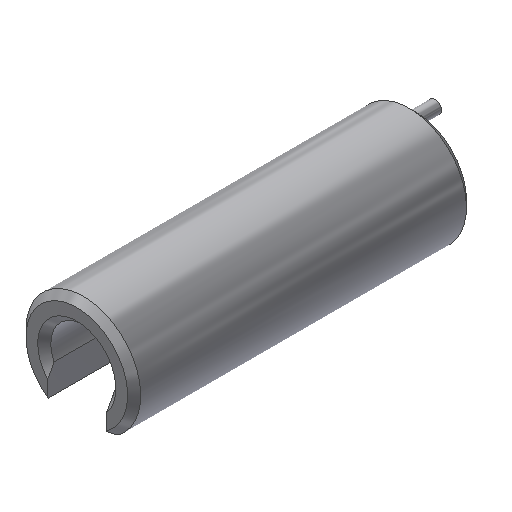
# Autodesk Inventor part: Adjustment tool
Saved by Autodesk Inventor 2022.4 (Build 264492000, 492)
## iProperties
Category: -
Company: Universiteit van Amsterdam
Created: 2023-09-04
Part Number: Adjustment tool
Material: ALMg4,5Mn-5083-(D54S)
Document SubType Name: Modeling
Designer: Ronald Hassing
Density: 2.66 g/cm^3
Appearance: Aluminum - Flat(2)
User Status: Work in Progress
Author: Ronald Hassing
Revision Number: A
Autodesk Inventor part; units mm, degrees
ref_plane "YZ Plane" through (0, 0, 0) normal (1, 0, 0) x (0, 1, 0)
ref_plane "XZ Plane" through (0, 0, 0) normal (0, 1, 0) x (-1, 0, 0)
ref_plane "XY Plane" through (0, 0, 0) normal (0, 0, 1) x (1, 0, 0)
sketch "Sketch1" plane through (0, 0, 0) normal (0, 0, 1) x (1, 0, 0)
  line L0 (0, 6.16) -> (0, -6.16) construction
  line L1 (-6.16, 0) -> (6.16, 0) construction
  circle A0 centre (0, 0) radius 4.4
  circle A1 centre (0, 0) radius 2.5
  circle A2 centre (0, 3.5) radius 0.5
  line L2 (-2.25, -1.0897) -> (-2.25, -3.7812)
  line L3 (2.25, -1.0897) -> (2.25, -3.7812)
  point P0 (-2.25, -2.4355)
  dimension "d4" = 8.8
  dimension "d5" = 5
  dimension "d6" = 3.5
  dimension "d7" = 1
  dimension "d16" = 4.5
  constraints: 4 end point, 4 point on circle, 3 centre point, 2 coincident, 1 horizontal alignment, 1 midpoint, 1 parallel, 1 point on line, 1 vertical
  measures "d4" diameter of A0
  measures "d5" diameter of A1
  measures "d6" distance of A2.centre point (0, 0)
  measures "d7" diameter of A2
  measures "d16" distance from line of L3 point (-2.25, -2.435)
extrude "Extrusion3" add sketch "Sketch1" along normal blind 26 contours A0 L3 A1 L2 | A2 picked at (-2.534, -2.6638)
extrude "Extrusion4" add sketch "Sketch1" against normal blind 1.5 contours A2
chamfer "Chamfer1" distance 0.5 angle 45 4 edges at (0, 4.4, 0) (0, 2.5, 0) (0, 2.5, 26) (0, 4.4, 26)
chamfer "Chamfer2" distance 0.5 angle 45 2 edges at (2.25, -3.7812, 13) (-2.25, -3.7812, 13)
body "Solid3"
